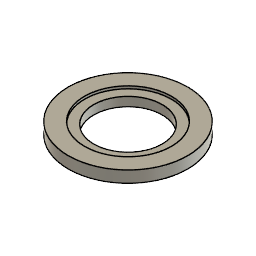
gearbox_ring (Autodesk Fusion 360 design; units mm, degrees)
Autodesk Fusion 360 part; units mm, degrees
sketch "Sketch1" plane through (0, 0, 0) normal (0, 1, 0) x (1, 0, 0)
  circle A0 centre (0, 0) radius 5
  circle A1 centre (0, 0) radius 2.5
  dimension "d1" = 10
  dimension "d2" = 5
  constraint coincident A0.centre A1.centre
  constraint concentric A0 A1
  measures "d1" diameter of A0
  measures "d2" diameter of A1
sketch "Sketch2" plane through (0, 0, 0) normal (0, 1, 0) x (1, 0, 0)
  circle A0 centre (0, 0) radius 5
  circle A1 centre (0, 0) radius 4
  dimension "d5" = 10
  dimension "d6" = 8
  constraint coincident A0.centre A1.centre
  measures "d5" diameter of A0
  measures "d6" diameter of A1
sketch "Sketch3" plane through (0, 0, 0) normal (0, 1, 0) x (1, 0, 0)
  circle A0 centre (0, 0) radius 5.15
  circle A1 centre (0, 0) radius 2.85
  dimension "d9" = 10.3
  dimension "d10" = 5.7
  constraint coincident A0.centre A1.centre
  measures "d9" diameter of A0
  measures "d10" diameter of A1
extrude "Extrude3" add sketch "Sketch3" along normal blind 1
move_face "OffsetFaces1" offset -0.05 1 faces at (2.8465, 0.6667, 0.1421)
sketch "Sketch4" plane through (0, 1, 0) normal (0, 1, 0) x (-1, 0, 0)
  circle A0 centre (0, 0) radius 2.9
  circle A1 centre (0, 0) radius 5.15
  circle A2 centre (0, 0) radius 3.4
  dimension "d14" = 6.8
  constraint concentric A0 A2
  measures "d14" diameter of A2
extrude "Extrude4" cut sketch "Sketch4" against normal blind 0.15 contours A2
move_face "OffsetFaces2" offset -0.1 1 faces at (2.8964, 0.5667, 0.1446)
move_face "OffsetFaces3" offset 0.05 1 faces at (2.9963, 0.2833, -0.1495)
move_face "OffsetFaces4" offset -0.07 1 faces at (-3.2264, 0.85, -0.3155)
move_face "OffsetFaces5" offset -0.05 1 faces at (-3.3958, 0.8533, -0.1695)
move_face "OffsetFaces6" offset -0.3 1 faces at (-3.4457, 0.8533, -0.172)
equation "d6 = 10 mm - 2 mm"
equation "d10 = 10.3 mm - ( 2.3 * 2 ) * 1 mm"
equation "d14 = 5.800 mm + 1 mm"
